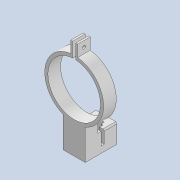
# Autodesk Inventor part: 0008-10-055 Doking
Saved by Autodesk Inventor 2020 (Build 240168000, 168)
## iProperties
Created: 2021-03-12
Part Number: 0008-10-055 Doking
Material: Generic
Document SubType Name: Modeling
Designer: Iulian Bors
Density: 1 g/cm^3
Appearance: Default
Description: Doking
Mass: 86.4445 g
Surface Area: 272.996 cm^2
Volume: 86.4445 cm^3
Author: Iulian Bors
Subject: 055
Autodesk Inventor part; units mm, degrees
ref_plane "YZ Plane" through (0, 0, 0) normal (1, 0, 0) x (0, 1, 0)
ref_plane "XZ Plane" through (0, 0, 0) normal (0, 1, 0) x (-1, 0, 0)
ref_plane "XY Plane" through (0, 0, 0) normal (0, 0, 1) x (1, 0, 0)
sketch "Sketch1" plane through (0, 0, 0) normal (0, 0, 1) x (1, 0, 0)
  arc A0 (-2.5, 41.4246) -> (2.5, 41.4246) centre (0, 0) ccw
  arc A1 (-5.5, 46.1736) -> (5.5, 46.1736) centre (0, 0) ccw
  line L0 (-2.5, 61.4493) -> (2.5, 61.4493)
  line L1 (2.5, 61.4493) -> (2.5, 41.4246)
  line L2 (-2.5, 41.4246) -> (-2.5, 61.4493)
  line L3 (5.5, 46.1736) -> (5.5, 64.4493)
  line L4 (-5.5, 64.4493) -> (-5.5, 46.1736)
  line L5 (-2.5, 61.4493) -> (-2.5, 64.4493)
  line L6 (2.5, 61.4493) -> (2.5, 64.4493)
  line L7 (5.5, 64.4493) -> (2.5, 64.4493)
  line L8 (-2.5, 64.4493) -> (-5.5, 64.4493)
  line L9 (-17.5, -41.5) -> (17.5, -41.5)
  line L10 (17.5, -41.5) -> (17.5, -91.5)
  line L11 (17.5, -91.5) -> (-17.5, -91.5)
  line L12 (-17.5, -91.5) -> (-17.5, -41.5)
  point P0 (0, 61.4493)
  point P1 (0, -91.5)
  point P2 (-17.5, -43.0813)
  point P3 (17.5, -43.0813)
  point P4 (16.5831, -25)
  point P5 (-16.5831, -25)
  point P6 (0, -41.5)
  dimension "d0" = 83
  dimension "d1" = 93
  dimension "d4" = 3
  dimension "d5" = 5
  dimension "d6" = 3
  dimension "d7" = 3
  dimension "d8" = 35
  dimension "d9" = 50
  dimension "d35" = 15.2757
  constraints: 26 end point, 8 perpendicular, 4 parallel, 4 point on circle, 2 centre point, 2 coincident, 2 horizontal, 2 midpoint, 2 vertical alignment, 1 collinear, 1 tangent
  measures "d0" diameter of A0
  measures "d1" diameter of A1
  measures "d4" distance between parallel lines of L1 L3
  measures "d5" distance between parallel lines of L1 L2
  measures "d6" distance of L5.end L4.start
  measures "d7" distance from line of point (0, 61.449) L8
  measures "d8" distance of L10.end L11.end
  measures "d9" distance of L11.end L9.start
  measures "d35" vertical distance of L4.end point (0, 61.449)
extrude "Extrusion1" add sketch "Sketch1" along normal blind 20 contours A0 L9 L12 A1 L4 L8 L5 L2 | L9 L10 A1 L12 | A0 L1 L6 L7 L3 A1 L10 L9 | A1 L10 L11 L12
sketch "Sketch2" plane through (5.5, 46.1736, 0) normal (1, 0, 0) x (0, 0, -1)
  line L0 (-20, 0) -> (-20, 18.2757) projected
  line L1 (0, 18.2757) -> (-20, 18.2757) projected
  point P0 (0, -46.1736)
  point P1 (-10, 9.1378)
  point P2 (-20, 9.1378)
  point P3 (-10, 18.2757)
  constraints: 2 midpoint, 1 horizontal alignment, 1 vertical alignment
hole "Hole1" at (5.5, 55.3114, 10) direction (-1, 0, 0) diameter 5 end through all
sketch "Sketch3" plane through (0, 0, 0) normal (0, 0, -1) x (-1, 0, 0)
  arc A0 (-5.5, 46.1736) -> (-17.5, -43.0813) centre (0, 0) ccw projected
  line L0 (5.5, 64.4493) -> (5.5, 46.1736) projected
  line L1 (2.5, 64.4493) -> (5.5, 64.4493) projected
  line L2 (2.5, 41.4246) -> (2.5, 64.4493) projected
  arc A1 (-2.5, 41.4246) -> (2.5, 41.4246) centre (0, 0) ccw projected
  line L3 (-2.5, 64.4493) -> (-2.5, 41.4246) projected
  line L4 (-5.5, 64.4493) -> (-2.5, 64.4493) projected
  line L5 (-5.5, 46.1736) -> (-5.5, 64.4493) projected
  arc A2 (-5.5, 46.1736) -> (-17.5, -43.0813) centre (0, 0) ccw projected
  arc A3 (17.5, -43.0813) -> (5.5, 46.1736) centre (0, 0) ccw projected
  line L6 (-17.5, -58.6416) -> (17.5, -58.6416)
  arc A4 (17.5, -43.0813) -> (5.5, 46.1736) centre (0, 0) ccw projected
  line L7 (-17.5, -91.5) -> (-17.5, -43.0813) projected
  line L8 (17.5, -91.5) -> (-17.5, -91.5) projected
  line L9 (17.5, -43.0813) -> (17.5, -91.5) projected
  point P0 (16.5831, -25)
  point P1 (-16.5831, -25)
  point P2 (17.5, -58.6416)
  point P3 (-17.5, -58.6416)
  dimension "d36" = 32.8584
  constraints: 2 end point, 1 horizontal
  measures "d36" distance between parallel lines of L8 L6
extrude "Extrusion2" add sketch "Sketch3" along normal blind 30 contours L6 L9 L8 L7
sketch "Sketch4" plane through (17.5, -91.5, 20) normal (1, 0, 0) x (0, 0, -1)
  line L0 (50, 32.8584) -> (20, 32.8584)
  line L1 (20, 32.8584) -> (20, 30)
  line L2 (20, 30) -> (50, 30)
  line L3 (50, 30) -> (50, 32.8584)
  line L4 (50, 0) -> (0, 0) projected
  line L5 (50, 32.8584) -> (50, 0) projected
  line L6 (20, 32.8584) -> (50, 32.8584) projected
  line L7 (20, 32.8584) -> (20, 48.4187) projected
  point P0 (20, 91.5)
  point P1 (20, 0)
  point P2 (20, 60)
  dimension "d22" = 30
  constraints: 8 end point, 3 collinear, 1 horizontal, 1 parallel
  measures "d22" distance between parallel lines of L4 L2
extrude "Extrusion3" cut sketch "Sketch4" against normal through all
sketch "Sketch6" plane through (-17.5, -91.5, 20) normal (0, -1, 0) x (1, 0, 0)
  line L0 (27.5, -35) -> (24.5, -35)
  line L1 (24.5, -35) -> (24.5, -40)
  line L2 (24.5, -40) -> (10.5, -40)
  line L3 (10.5, -40) -> (10.5, -35)
  line L4 (10.5, -35) -> (7.5, -35)
  line L5 (7.5, -35) -> (7.5, -20)
  line L6 (7.5, -20) -> (27.5, -20)
  line L7 (27.5, -20) -> (27.5, -35)
  line L8 (27.75, -19.75) -> (7.25, -19.75)
  line L9 (7.25, -19.75) -> (7.25, -35.25)
  line L10 (7.25, -35.25) -> (10.25, -35.25)
  line L11 (10.25, -35.25) -> (10.25, -40.25)
  line L12 (10.25, -40.25) -> (24.75, -40.25)
  line L13 (24.75, -40.25) -> (24.75, -35.25)
  line L14 (24.75, -35.25) -> (27.75, -35.25)
  line L15 (27.75, -35.25) -> (27.75, -19.75)
  point P0 (17.5, -20)
  dimension "d28" = 0.25
  constraints: 32 end point, 4 horizontal, 4 vertical, 15 other
  measures "d28" distance between parallel lines of L6 L8
extrude "Extrusion5" cut sketch "Sketch6" against normal through all contours L0 L1 L2 L3 L4 L5 L6 L7 | L15 L14 L13 L12 L11 L10 L9 L8
sketch "Sketch9" plane through (10.25, -91.5, -15.25) normal (-1, 0, 0) x (0, 0, 1)
  line L0 (10.25, 30) -> (5.25, 30)
  line L1 (5.25, 30) -> (5.25, 10)
  line L2 (5.25, 10) -> (10.25, 10)
  line L3 (10.25, 10) -> (10.25, 30)
  line L4 (0, 30) -> (15.25, 30) projected
  line L5 (15.5, 0) -> (0, 0) projected
  point P0 (15.25, 91.5)
  point P1 (7.75, 10)
  point P2 (7.75, 0)
  point P3 (15.5, 25)
  dimension "d31" = 5
  dimension "d32" = 20
  constraints: 8 end point, 2 parallel, 1 collinear, 1 horizontal, 1 midpoint, 1 perpendicular, 1 vertical alignment, 2 other
  measures "d31" distance of L0.start L0.end
  measures "d32" distance of L2.end L0.start
extrude "Extrusion6" cut sketch "Sketch9" against normal through all
chamfer "Chamfer1" distance 2 angle 45 2 edges at (-17.5, -61.5, -15) (17.5, -61.5, -20)
body "Solid1"
